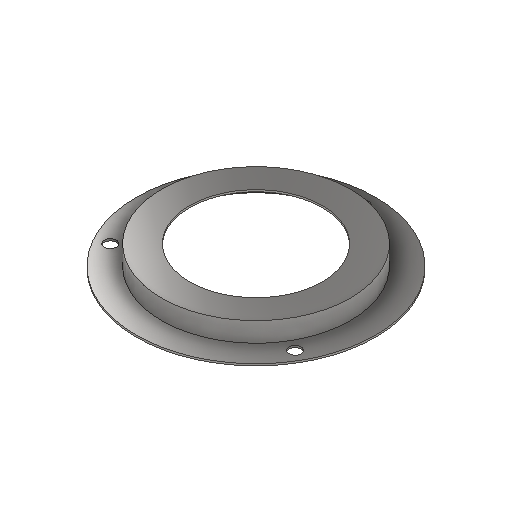
# Autodesk Inventor part: clamp_for_bearing
Saved by Autodesk Inventor 2026.2 (Build 302298000, 298)
## iProperties
Created: 2026-07-16
Part Number: clamp_for_bearing
Material: ステンレス鋼
Document SubType Name: Modeling
Designer: zetsu
Density: 8 g/cm^3
Appearance: 半つや出し
Author: zetsu
Autodesk Inventor part; units mm, degrees
ref_plane "YZ Plane" through (0, 0, 0) normal (1, 0, 0) x (0, 1, 0)
ref_plane "XZ Plane" through (0, 0, 0) normal (0, 1, 0) x (-1, 0, 0)
ref_plane "XY Plane" through (0, 0, 0) normal (0, 0, 1) x (1, 0, 0)
sketch "スケッチ1" plane through (0, 0, 0) normal (0, 1, 0) x (-1, 0, 0)
  circle A0 centre (0, 0) radius 32.5
  dimension "d0" = 65
  constraints: 1 centre point, 1 coincident
  measures "d0" diameter of A0
extrude "押し出し1" add sketch "スケッチ1" along normal blind 5.8
sketch "スケッチ2" plane through (0, 5.8, 0) normal (0, 1, 0) x (1, 0, 0)
  circle A0 centre (0, 0) radius 18
  dimension "d3" = 36
  constraints: 1 centre point, 1 coincident
  measures "d3" diameter of A0
extrude "押し出し2" cut sketch "スケッチ2" against normal through all
sketch "スケッチ3" plane through (0, 0, 0) normal (0, -1, 0) x (1, 0, 0)
  circle A0 centre (0, 0) radius 25.15
  dimension "d6" = 50.3
  constraints: 1 centre point, 1 coincident
  measures "d6" diameter of A0
extrude "押し出し3" cut sketch "スケッチ3" against normal blind 5.3
sketch "スケッチ4" plane through (0, 5.8, 0) normal (0, 1, 0) x (1, 0, 0)
  circle A0 centre (0, 0) radius 32.5
  circle A1 centre (0, 0) radius 25.65
  dimension "d9" = 51.3
  constraints: 2 centre point, 2 coincident
  measures "d9" diameter of A1
extrude "押し出し4" cut sketch "スケッチ4" against normal blind 5.3
sketch "スケッチ5" plane through (0, 0.5, 0) normal (0, 1, 0) x (1, 0, 0)
  circle A0 centre (0, 29) radius 1.65
  circle A1 centre (-25.1147, -14.5) radius 1.65
  circle A2 centre (25.1147, -14.5) radius 1.65
  point P0 (0, 0)
  dimension "d12" = 3.3
  dimension "d13" = 29
  dimension "d16" = 360
  constraints: 3 centre point, 7 other
  measures "d12" diameter of A0
  measures "d13" distance of point (0, 0) A0.centre
extrude "押し出し5" cut sketch "スケッチ5" against normal through all
